Autodesk Fusion 360 part; units mm, degrees
(part 4 of 5)
sketch "Sketch1 (2)" plane through (0, 0, 25) normal (0, 0, 1) x (-1, 0, 0)
  arc A0 (-16.5263, 3.7625) -> (-16.7082, 2.8483) centre (0, 0) ccw
  arc A1 (-17.8062, 2.0227) -> (-16.7082, 2.8483) centre (-17.6939, 3.0163) ccw
  line L0 (-17.8062, 2.0227) -> (-18.6738, 2.1207)
  spline S0 degree 5 poles (-18.6738, 2.1207) (-18.6847, 2.1219) (-18.7065, 2.124) (-18.7393, 2.1263) (-18.783, 2.1276) (-18.8378, 2.1268) (-18.8928, 2.1242) (-18.9478, 2.1205) (-19.0028, 2.1162) (-19.0579, 2.1115) (-19.113, 2.1064) (-19.1681, 2.1008) (-19.2232, 2.0944) (-19.2784, 2.0871) (-19.3336, 2.079) (-19.3888, 2.0701) (-19.444, 2.0605) (-19.4992, 2.0503) (-19.5544, 2.0396) (-19.6096, 2.0285) (-19.6648, 2.0169) (-19.72, 2.0048) (-19.7752, 1.9921) (-19.8303, 1.9789) (-19.8855, 1.9652) (-19.9406, 1.9509) (-19.9957, 1.9362) (-20.0508, 1.921) (-20.1059, 1.9054) (-20.1609, 1.8893) (-20.2159, 1.8728) (-20.2709, 1.8558) (-20.3259, 1.8384) (-20.3808, 1.8206) (-20.4357, 1.8024) (-20.4906, 1.7837) (-20.5454, 1.7646) (-20.6002, 1.7451) (-20.655, 1.7252) (-20.7097, 1.7049) (-20.7643, 1.6842) (-20.819, 1.6631) (-20.8736, 1.6416) (-20.9281, 1.6198) (-20.9826, 1.5975) (-21.037, 1.5749) (-21.0914, 1.5519) (-21.1458, 1.5285) (-21.2001, 1.5048) (-21.2543, 1.4807) (-21.3085, 1.4563) (-21.3626, 1.4315) (-21.4167, 1.4063) (-21.4707, 1.3808) (-21.5247, 1.3549) (-21.5786, 1.3287) (-21.6324, 1.3021) (-21.6862, 1.2752) (-21.7399, 1.248) (-21.7936, 1.2204) (-21.8471, 1.1925) (-21.9007, 1.1642) (-21.9541, 1.1356) (-22.0075, 1.1067) (-22.0608, 1.0775) (-22.114, 1.0479) (-22.1672, 1.018) (-22.2203, 0.9878) (-22.2733, 0.9573) (-22.3263, 0.9265) (-22.3791, 0.8953) (-22.4214, 0.8701) (-22.453, 0.8511) (-22.4741, 0.8383) (-22.4846, 0.8319) knots 0 0 0 0 0 0 0.01428571 0.02857143 0.04285714 0.05714286 0.07142857 0.08571429 0.1 0.11428571 0.12857143 0.14285714 0.15714286 0.17142857 0.18571429 0.2 0.21428571 0.22857143 0.24285714 0.25714286 0.27142857 0.28571429 0.3 0.31428571 0.32857143 0.34285714 0.35714286 0.37142857 0.38571429 0.4 0.41428571 0.42857143 0.44285714 0.45714286 0.47142857 0.48571429 0.5 0.51428571 0.52857143 0.54285714 0.55714286 0.57142857 0.58571429 0.6 0.61428571 0.62857143 0.64285714 0.65714286 0.67142857 0.68571429 0.7 0.71428571 0.72857143 0.74285714 0.75714286 0.77142857 0.78571429 0.8 0.81428571 0.82857143 0.84285714 0.85714286 0.87142857 0.88571429 0.9 0.91428571 0.92857143 0.94285714 0.95714286 0.97142857 0.98571429 1 1 1 1 1 1
  arc A2 (-22.4846, 0.8319) -> (-22.4846, -0.8319) centre (0, 0) ccw
  spline S1 degree 5 poles (-22.4846, -0.8319) (-22.4741, -0.8383) (-22.453, -0.8511) (-22.4214, -0.8701) (-22.3791, -0.8953) (-22.3263, -0.9265) (-22.2733, -0.9573) (-22.2203, -0.9878) (-22.1672, -1.018) (-22.114, -1.0479) (-22.0608, -1.0775) (-22.0075, -1.1067) (-21.9541, -1.1356) (-21.9007, -1.1642) (-21.8471, -1.1925) (-21.7936, -1.2204) (-21.7399, -1.248) (-21.6862, -1.2752) (-21.6324, -1.3021) (-21.5786, -1.3287) (-21.5247, -1.3549) (-21.4707, -1.3808) (-21.4167, -1.4063) (-21.3626, -1.4315) (-21.3085, -1.4563) (-21.2543, -1.4807) (-21.2001, -1.5048) (-21.1458, -1.5285) (-21.0914, -1.5519) (-21.037, -1.5749) (-20.9826, -1.5975) (-20.9281, -1.6198) (-20.8736, -1.6416) (-20.819, -1.6631) (-20.7643, -1.6842) (-20.7097, -1.7049) (-20.655, -1.7252) (-20.6002, -1.7451) (-20.5454, -1.7646) (-20.4906, -1.7837) (-20.4357, -1.8024) (-20.3808, -1.8206) (-20.3259, -1.8384) (-20.2709, -1.8558) (-20.2159, -1.8728) (-20.1609, -1.8893) (-20.1059, -1.9054) (-20.0508, -1.921) (-19.9957, -1.9362) (-19.9406, -1.9509) (-19.8855, -1.9652) (-19.8303, -1.9789) (-19.7752, -1.9921) (-19.72, -2.0048) (-19.6648, -2.0169) (-19.6096, -2.0285) (-19.5544, -2.0396) (-19.4992, -2.0503) (-19.444, -2.0605) (-19.3888, -2.0701) (-19.3336, -2.079) (-19.2784, -2.0871) (-19.2232, -2.0944) (-19.1681, -2.1008) (-19.113, -2.1064) (-19.0579, -2.1115) (-19.0028, -2.1162) (-18.9478, -2.1205) (-18.8928, -2.1242) (-18.8378, -2.1268) (-18.783, -2.1276) (-18.7393, -2.1263) (-18.7065, -2.124) (-18.6847, -2.1219) (-18.6738, -2.1207) knots -1 -1 -1 -1 -1 -1 -0.98571429 -0.97142857 -0.95714286 -0.94285714 -0.92857143 -0.91428571 -0.9 -0.88571429 -0.87142857 -0.85714286 -0.84285714 -0.82857143 -0.81428571 -0.8 -0.78571429 -0.77142857 -0.75714286 -0.74285714 -0.72857143 -0.71428571 -0.7 -0.68571429 -0.67142857 -0.65714286 -0.64285714 -0.62857143 -0.61428571 -0.6 -0.58571429 -0.57142857 -0.55714286 -0.54285714 -0.52857143 -0.51428571 -0.5 -0.48571429 -0.47142857 -0.45714286 -0.44285714 -0.42857143 -0.41428571 -0.4 -0.38571429 -0.37142857 -0.35714286 -0.34285714 -0.32857143 -0.31428571 -0.3 -0.28571429 -0.27142857 -0.25714286 -0.24285714 -0.22857143 -0.21428571 -0.2 -0.18571429 -0.17142857 -0.15714286 -0.14285714 -0.12857143 -0.11428571 -0.1 -0.08571429 -0.07142857 -0.05714286 -0.04285714 -0.02857143 -0.01428571 0 0 0 0 0 0
  line L1 (-18.6738, -2.1207) -> (-17.8062, -2.0227)
  arc A3 (-16.7082, -2.8483) -> (-17.8062, -2.0227) centre (-17.6939, -3.0163) ccw
  arc A4 (-16.7082, -2.8483) -> (-16.5263, -3.7625) centre (0, 0) ccw
  arc A5 (-17.2248, -4.9454) -> (-16.5263, -3.7625) centre (-17.5014, -3.9844) ccw
  line L2 (-17.2248, -4.9454) -> (-18.0639, -5.1869)
  spline S2 degree 5 poles (-18.0639, -5.1869) (-18.0744, -5.19) (-18.0954, -5.1963) (-18.1265, -5.2067) (-18.1674, -5.2223) (-18.2178, -5.2441) (-18.2675, -5.2675) (-18.3169, -5.2919) (-18.3661, -5.3169) (-18.4152, -5.3423) (-18.4642, -5.3681) (-18.5129, -5.3944) (-18.5614, -5.4215) (-18.6096, -5.4493) (-18.6575, -5.4779) (-18.7051, -5.5073) (-18.7524, -5.5373) (-18.7995, -5.5678) (-18.8464, -5.5988) (-18.8932, -5.6302) (-18.9397, -5.662) (-18.9861, -5.6944) (-19.0322, -5.7272) (-19.0781, -5.7605) (-19.1238, -5.7942) (-19.1693, -5.8285) (-19.2146, -5.8632) (-19.2597, -5.8983) (-19.3046, -5.9338) (-19.3493, -5.9698) (-19.3938, -6.0061) (-19.4381, -6.0428) (-19.4822, -6.0799) (-19.5261, -6.1174) (-19.5699, -6.1552) (-19.6134, -6.1935) (-19.6568, -6.2321) (-19.6999, -6.2711) (-19.7429, -6.3105) (-19.7857, -6.3502) (-19.8283, -6.3902) (-19.8707, -6.4306) (-19.9129, -6.4713) (-19.9549, -6.5124) (-19.9967, -6.5538) (-20.0384, -6.5955) (-20.0798, -6.6376) (-20.1211, -6.68) (-20.1622, -6.7227) (-20.2031, -6.7657) (-20.2438, -6.809) (-20.2843, -6.8526) (-20.3246, -6.8966) (-20.3648, -6.9408) (-20.4047, -6.9854) (-20.4445, -7.0302) (-20.484, -7.0754) (-20.5234, -7.1208) (-20.5626, -7.1665) (-20.6016, -7.2125) (-20.6405, -7.2588) (-20.6791, -7.3054) (-20.7175, -7.3523) (-20.7558, -7.3994) (-20.7939, -7.4468) (-20.8317, -7.4945) (-20.8694, -7.5425) (-20.9069, -7.5907) (-20.9442, -7.6392) (-20.9813, -7.688) (-21.0182, -7.737) (-21.0476, -7.7764) (-21.0696, -7.8061) (-21.0842, -7.8259) (-21.0914, -7.8359) knots 0 0 0 0 0 0 0.01428571 0.02857143 0.04285714 0.05714286 0.07142857 0.08571429 0.1 0.11428571 0.12857143 0.14285714 0.15714286 0.17142857 0.18571429 0.2 0.21428571 0.22857143 0.24285714 0.25714286 0.27142857 0.28571429 0.3 0.31428571 0.32857143 0.34285714 0.35714286 0.37142857 0.38571429 0.4 0.41428571 0.42857143 0.44285714 0.45714286 0.47142857 0.48571429 0.5 0.51428571 0.52857143 0.54285714 0.55714286 0.57142857 0.58571429 0.6 0.61428571 0.62857143 0.64285714 0.65714286 0.67142857 0.68571429 0.7 0.71428571 0.72857143 0.74285714 0.75714286 0.77142857 0.78571429 0.8 0.81428571 0.82857143 0.84285714 0.85714286 0.87142857 0.88571429 0.9 0.91428571 0.92857143 0.94285714 0.95714286 0.97142857 0.98571429 1 1 1 1 1 1
  arc A6 (-21.0914, -7.8359) -> (-20.4547, -9.3731) centre (0, 0) ccw
  spline S3 degree 5 poles (-20.4547, -9.3731) (-20.4425, -9.375) (-20.4182, -9.3787) (-20.3817, -9.3842) (-20.333, -9.3913) (-20.2722, -9.3998) (-20.2115, -9.4081) (-20.1508, -9.416) (-20.0902, -9.4236) (-20.0297, -9.4308) (-19.9692, -9.4378) (-19.9087, -9.4444) (-19.8484, -9.4507) (-19.788, -9.4566) (-19.7278, -9.4622) (-19.6676, -9.4675) (-19.6075, -9.4725) (-19.5474, -9.4771) (-19.4874, -9.4814) (-19.4275, -9.4853) (-19.3677, -9.4889) (-19.308, -9.4922) (-19.2483, -9.4951) (-19.1887, -9.4976) (-19.1292, -9.4998) (-19.0698, -9.5017) (-19.0104, -9.5032) (-18.9512, -9.5043) (-18.8921, -9.5051) (-18.833, -9.5055) (-18.774, -9.5056) (-18.7152, -9.5053) (-18.6564, -9.5046) (-18.5978, -9.5036) (-18.5392, -9.5021) (-18.4808, -9.5003) (-18.4225, -9.4982) (-18.3643, -9.4956) (-18.3062, -9.4926) (-18.2482, -9.4893) (-18.1904, -9.4856) (-18.1327, -9.4814) (-18.0751, -9.4769) (-18.0177, -9.4719) (-17.9604, -9.4665) (-17.9033, -9.4607) (-17.8462, -9.4545) (-17.7894, -9.4479) (-17.7327, -9.4409) (-17.6761, -9.4334) (-17.6197, -9.4254) (-17.5635, -9.417) (-17.5075, -9.4081) (-17.4517, -9.3987) (-17.3961, -9.3887) (-17.3406, -9.3784) (-17.2854, -9.3675) (-17.2303, -9.3563) (-17.1754, -9.3445) (-17.1207, -9.3323) (-17.0663, -9.3194) (-17.0122, -9.3058) (-16.9585, -9.2914) (-16.9051, -9.2762) (-16.852, -9.2603) (-16.7991, -9.2439) (-16.7465, -9.2272) (-16.694, -9.2101) (-16.6417, -9.1924) (-16.59, -9.1738) (-16.539, -9.1536) (-16.4991, -9.1357) (-16.4697, -9.121) (-16.4504, -9.1107) (-16.4408, -9.1054) knots -1 -1 -1 -1 -1 -1 -0.98571429 -0.97142857 -0.95714286 -0.94285714 -0.92857143 -0.91428571 -0.9 -0.88571429 -0.87142857 -0.85714286 -0.84285714 -0.82857143 -0.81428571 -0.8 -0.78571429 -0.77142857 -0.75714286 -0.74285714 -0.72857143 -0.71428571 -0.7 -0.68571429 -0.67142857 -0.65714286 -0.64285714 -0.62857143 -0.61428571 -0.6 -0.58571429 -0.57142857 -0.55714286 -0.54285714 -0.52857143 -0.51428571 -0.5 -0.48571429 -0.47142857 -0.45714286 -0.44285714 -0.42857143 -0.41428571 -0.4 -0.38571429 -0.37142857 -0.35714286 -0.34285714 -0.32857143 -0.31428571 -0.3 -0.28571429 -0.27142857 -0.25714286 -0.24285714 -0.22857143 -0.21428571 -0.2 -0.18571429 -0.17142857 -0.15714286 -0.14285714 -0.12857143 -0.11428571 -0.1 -0.08571429 -0.07142857 -0.05714286 -0.04285714 -0.02857143 -0.01428571 0 0 0 0 0 0
  line L3 (-16.4408, -9.1054) -> (-15.6767, -8.6828)
  arc A7 (-14.3463, -9.0254) -> (-15.6767, -8.6828) centre (-15.1928, -9.5579) ccw
  arc A8 (-14.3463, -9.0254) -> (-13.8285, -9.8004) centre (0, 0) ccw
  arc A9 (-14.0211, -11.1606) -> (-13.8285, -9.8004) centre (-14.6444, -10.3786) ccw
  line L4 (-14.0211, -11.1606) -> (-14.7039, -11.7048)
  spline S4 degree 5 poles (-14.7039, -11.7048) (-14.7125, -11.7117) (-14.7294, -11.7256) (-14.7542, -11.7471) (-14.786, -11.7771) (-14.8242, -11.8165) (-14.8612, -11.8572) (-14.8975, -11.8987) (-14.9334, -11.9406) (-14.969, -11.9829) (-15.0044, -12.0254) (-15.0394, -12.0684) (-15.0738, -12.1119) (-15.1077, -12.1561) (-15.141, -12.2008) (-15.1737, -12.2462) (-15.206, -12.292) (-15.2378, -12.3382) (-15.2693, -12.3848) (-15.3004, -12.4317) (-15.3313, -12.479) (-15.3617, -12.5266) (-15.3918, -12.5745) (-15.4215, -12.6229) (-15.4507, -12.6716) (-15.4797, -12.7206) (-15.5082, -12.77) (-15.5364, -12.8197) (-15.5643, -12.8697) (-15.5919, -12.92) (-15.6191, -12.9706) (-15.646, -13.0214) (-15.6725, -13.0726) (-15.6988, -13.124) (-15.7247, -13.1758) (-15.7503, -13.2278) (-15.7755, -13.2801) (-15.8005, -13.3326) (-15.8251, -13.3854) (-15.8495, -13.4384) (-15.8735, -13.4917) (-15.8972, -13.5453) (-15.9206, -13.599) (-15.9437, -13.6531) (-15.9665, -13.7073) (-15.989, -13.7618) (-16.0113, -13.8165) (-16.0332, -13.8715) (-16.0548, -13.9267) (-16.0761, -13.982) (-16.0971, -14.0376) (-16.1179, -14.0935) (-16.1383, -14.1495) (-16.1584, -14.2057) (-16.1783, -14.2622) (-16.1979, -14.3188) (-16.2172, -14.3757) (-16.2362, -14.4327) (-16.2549, -14.49) (-16.2733, -14.5474) (-16.2915, -14.605) (-16.3093, -14.6629) (-16.3269, -14.7209) (-16.3442, -14.7791) (-16.3612, -14.8374) (-16.378, -14.896) (-16.3944, -14.9547) (-16.4106, -15.0136) (-16.4265, -15.0727) (-16.4421, -15.1319) (-16.4575, -15.1914) (-16.4696, -15.239) (-16.4785, -15.2749) (-16.4844, -15.2988) (-16.4873, -15.3108) knots 0 0 0 0 0 0 0.01428571 0.02857143 0.04285714 0.05714286 0.07142857 0.08571429 0.1 0.11428571 0.12857143 0.14285714 0.15714286 0.17142857 0.18571429 0.2 0.21428571 0.22857143 0.24285714 0.25714286 0.27142857 0.28571429 0.3 0.31428571 0.32857143 0.34285714 0.35714286 0.37142857 0.38571429 0.4 0.41428571 0.42857143 0.44285714 0.45714286 0.47142857 0.48571429 0.5 0.51428571 0.52857143 0.54285714 0.55714286 0.57142857 0.58571429 0.6 0.61428571 0.62857143 0.64285714 0.65714286 0.67142857 0.68571429 0.7 0.71428571 0.72857143 0.74285714 0.75714286 0.77142857 0.78571429 0.8 0.81428571 0.82857143 0.84285714 0.85714286 0.87142857 0.88571429 0.9 0.91428571 0.92857143 0.94285714 0.95714286 0.97142857 0.98571429 1 1 1 1 1 1
  arc A10 (-16.4873, -15.3108) -> (-15.3108, -16.4873) centre (0, 0) ccw
  spline S5 degree 5 poles (-15.3108, -16.4873) (-15.2988, -16.4844) (-15.2749, -16.4785) (-15.239, -16.4696) (-15.1914, -16.4575) (-15.1319, -16.4421) (-15.0727, -16.4265) (-15.0136, -16.4106) (-14.9547, -16.3944) (-14.896, -16.378) (-14.8374, -16.3612) (-14.7791, -16.3442) (-14.7209, -16.3269) (-14.6629, -16.3093) (-14.605, -16.2915) (-14.5474, -16.2733) (-14.49, -16.2549) (-14.4327, -16.2362) (-14.3757, -16.2172) (-14.3188, -16.1979) (-14.2622, -16.1783) (-14.2057, -16.1584) (-14.1495, -16.1383) (-14.0935, -16.1179) (-14.0376, -16.0971) (-13.982, -16.0761) (-13.9267, -16.0548) (-13.8715, -16.0332) (-13.8165, -16.0113) (-13.7618, -15.989) (-13.7073, -15.9665) (-13.6531, -15.9437) (-13.599, -15.9206) (-13.5453, -15.8972) (-13.4917, -15.8735) (-13.4384, -15.8495) (-13.3854, -15.8251) (-13.3326, -15.8005) (-13.2801, -15.7755) (-13.2278, -15.7503) (-13.1758, -15.7247) (-13.124, -15.6988) (-13.0726, -15.6725) (-13.0214, -15.646) (-12.9706, -15.6191) (-12.92, -15.5919) (-12.8697, -15.5643) (-12.8197, -15.5364) (-12.77, -15.5082) (-12.7206, -15.4797) (-12.6716, -15.4507) (-12.6229, -15.4215) (-12.5745, -15.3918) (-12.5266, -15.3617) (-12.479, -15.3313) (-12.4317, -15.3004) (-12.3848, -15.2693) (-12.3382, -15.2378) (-12.292, -15.206) (-12.2462, -15.1737) (-12.2008, -15.141) (-12.1561, -15.1077) (-12.1119, -15.0738) (-12.0684, -15.0394) (-12.0254, -15.0044) (-11.9829, -14.969) (-11.9406, -14.9334) (-11.8987, -14.8975) (-11.8572, -14.8612) (-11.8165, -14.8242) (-11.7771, -14.786) (-11.7471, -14.7542) (-11.7256, -14.7294) (-11.7117, -14.7125) (-11.7048, -14.7039) knots -1 -1 -1 -1 -1 -1 -0.98571429 -0.97142857 -0.95714286 -0.94285714 -0.92857143 -0.91428571 -0.9 -0.88571429 -0.87142857 -0.85714286 -0.84285714 -0.82857143 -0.81428571 -0.8 -0.78571429 -0.77142857 -0.75714286 -0.74285714 -0.72857143 -0.71428571 -0.7 -0.68571429 -0.67142857 -0.65714286 -0.64285714 -0.62857143 -0.61428571 -0.6 -0.58571429 -0.57142857 -0.55714286 -0.54285714 -0.52857143 -0.51428571 -0.5 -0.48571429 -0.47142857 -0.45714286 -0.44285714 -0.42857143 -0.41428571 -0.4 -0.38571429 -0.37142857 -0.35714286 -0.34285714 -0.32857143 -0.31428571 -0.3 -0.28571429 -0.27142857 -0.25714286 -0.24285714 -0.22857143 -0.21428571 -0.2 -0.18571429 -0.17142857 -0.15714286 -0.14285714 -0.12857143 -0.11428571 -0.1 -0.08571429 -0.07142857 -0.05714286 -0.04285714 -0.02857143 -0.01428571 0 0 0 0 0 0
  line L5 (-11.7048, -14.7039) -> (-11.1606, -14.0211)
  arc A11 (-9.8004, -13.8285) -> (-11.1606, -14.0211) centre (-10.3786, -14.6444) ccw
  arc A12 (-9.8004, -13.8285) -> (-9.0254, -14.3463) centre (0, 0) ccw
  arc A13 (-8.6828, -15.6767) -> (-9.0254, -14.3463) centre (-9.5579, -15.1928) ccw
  line L6 (-8.6828, -15.6767) -> (-9.1054, -16.4408)
  spline S6 degree 5 poles (-9.1054, -16.4408) (-9.1107, -16.4504) (-9.121, -16.4697) (-9.1357, -16.4991) (-9.1536, -16.539) (-9.1738, -16.59) (-9.1924, -16.6417) (-9.2101, -16.694) (-9.2272, -16.7465) (-9.2439, -16.7991) (-9.2603, -16.852) (-9.2762, -16.9051) (-9.2914, -16.9585) (-9.3058, -17.0122) (-9.3194, -17.0663) (-9.3323, -17.1207) (-9.3445, -17.1754) (-9.3563, -17.2303) (-9.3675, -17.2854) (-9.3784, -17.3406) (-9.3887, -17.3961) (-9.3987, -17.4517) (-9.4081, -17.5075) (-9.417, -17.5635) (-9.4254, -17.6197) (-9.4334, -17.6761) (-9.4409, -17.7327) (-9.4479, -17.7894) (-9.4545, -17.8462) (-9.4607, -17.9033) (-9.4665, -17.9604) (-9.4719, -18.0177) (-9.4769, -18.0751) (-9.4814, -18.1327) (-9.4856, -18.1904) (-9.4893, -18.2482) (-9.4926, -18.3062) (-9.4956, -18.3643) (-9.4982, -18.4225) (-9.5003, -18.4808) (-9.5021, -18.5392) (-9.5036, -18.5978) (-9.5046, -18.6564) (-9.5053, -18.7152) (-9.5056, -18.774) (-9.5055, -18.833) (-9.5051, -18.8921) (-9.5043, -18.9512) (-9.5032, -19.0104) (-9.5017, -19.0698) (-9.4998, -19.1292) (-9.4976, -19.1887) (-9.4951, -19.2483) (-9.4922, -19.308) (-9.4889, -19.3677) (-9.4853, -19.4275) (-9.4814, -19.4874) (-9.4771, -19.5474) (-9.4725, -19.6075) (-9.4675, -19.6676) (-9.4622, -19.7278) (-9.4566, -19.788) (-9.4507, -19.8484) (-9.4444, -19.9087) (-9.4378, -19.9692) (-9.4308, -20.0297) (-9.4236, -20.0902) (-9.416, -20.1508) (-9.4081, -20.2115) (-9.3998, -20.2722) (-9.3913, -20.333) (-9.3842, -20.3817) (-9.3787, -20.4182) (-9.375, -20.4425) (-9.3731, -20.4547) knots 0 0 0 0 0 0 0.01428571 0.02857143 0.04285714 0.05714286 0.07142857 0.08571429 0.1 0.11428571 0.12857143 0.14285714 0.15714286 0.17142857 0.18571429 0.2 0.21428571 0.22857143 0.24285714 0.25714286 0.27142857 0.28571429 0.3 0.31428571 0.32857143 0.34285714 0.35714286 0.37142857 0.38571429 0.4 0.41428571 0.42857143 0.44285714 0.45714286 0.47142857 0.48571429 0.5 0.51428571 0.52857143 0.54285714 0.55714286 0.57142857 0.58571429 0.6 0.61428571 0.62857143 0.64285714 0.65714286 0.67142857 0.68571429 0.7 0.71428571 0.72857143 0.74285714 0.75714286 0.77142857 0.78571429 0.8 0.81428571 0.82857143 0.84285714 0.85714286 0.87142857 0.88571429 0.9 0.91428571 0.92857143 0.94285714 0.95714286 0.97142857 0.98571429 1 1 1 1 1 1
  arc A14 (-9.3731, -20.4547) -> (-7.8359, -21.0914) centre (0, 0) ccw
  spline S7 degree 5 poles (-7.8359, -21.0914) (-7.8259, -21.0842) (-7.8061, -21.0696) (-7.7764, -21.0476) (-7.737, -21.0182) (-7.688, -20.9813) (-7.6392, -20.9442) (-7.5907, -20.9069) (-7.5425, -20.8694) (-7.4945, -20.8317) (-7.4468, -20.7939) (-7.3994, -20.7558) (-7.3523, -20.7175) (-7.3054, -20.6791) (-7.2588, -20.6405) (-7.2125, -20.6016) (-7.1665, -20.5626) (-7.1208, -20.5234) (-7.0754, -20.484) (-7.0302, -20.4445) (-6.9854, -20.4047) (-6.9408, -20.3648) (-6.8966, -20.3246) (-6.8526, -20.2843) (-6.809, -20.2438) (-6.7657, -20.2031) (-6.7227, -20.1622) (-6.68, -20.1211) (-6.6376, -20.0798) (-6.5955, -20.0384) (-6.5538, -19.9967) (-6.5124, -19.9549) (-6.4713, -19.9129) (-6.4306, -19.8707) (-6.3902, -19.8283) (-6.3502, -19.7857) (-6.3105, -19.7429) (-6.2711, -19.6999) (-6.2321, -19.6568) (-6.1935, -19.6134) (-6.1552, -19.5699) (-6.1174, -19.5261) (-6.0799, -19.4822) (-6.0428, -19.4381) (-6.0061, -19.3938) (-5.9698, -19.3493) (-5.9338, -19.3046) (-5.8983, -19.2597) (-5.8632, -19.2146) (-5.8285, -19.1693) (-5.7942, -19.1238) (-5.7605, -19.0781) (-5.7272, -19.0322) (-5.6944, -18.9861) (-5.662, -18.9397) (-5.6302, -18.8932) (-5.5988, -18.8464) (-5.5678, -18.7995) (-5.5373, -18.7524) (-5.5073, -18.7051) (-5.4779, -18.6575) (-5.4493, -18.6096) (-5.4215, -18.5614) (-5.3944, -18.5129) (-5.3681, -18.4642) (-5.3423, -18.4152) (-5.3169, -18.3661) (-5.2919, -18.3169) (-5.2675, -18.2675) (-5.2441, -18.2178) (-5.2223, -18.1674) (-5.2067, -18.1265) (-5.1963, -18.0954) (-5.19, -18.0744) (-5.1869, -18.0639) knots -1 -1 -1 -1 -1 -1 -0.98571429 -0.97142857 -0.95714286 -0.94285714 -0.92857143 -0.91428571 -0.9 -0.88571429 -0.87142857 -0.85714286 -0.84285714 -0.82857143 -0.81428571 -0.8 -0.78571429 -0.77142857 -0.75714286 -0.74285714 -0.72857143 -0.71428571 -0.7 -0.68571429 -0.67142857 -0.65714286 -0.64285714 -0.62857143 -0.61428571 -0.6 -0.58571429 -0.57142857 -0.55714286 -0.54285714 -0.52857143 -0.51428571 -0.5 -0.48571429 -0.47142857 -0.45714286 -0.44285714 -0.42857143 -0.41428571 -0.4 -0.38571429 -0.37142857 -0.35714286 -0.34285714 -0.32857143 -0.31428571 -0.3 -0.28571429 -0.27142857 -0.25714286 -0.24285714 -0.22857143 -0.21428571 -0.2 -0.18571429 -0.17142857 -0.15714286 -0.14285714 -0.12857143 -0.11428571 -0.1 -0.08571429 -0.07142857 -0.05714286 -0.04285714 -0.02857143 -0.01428571 0 0 0 0 0 0
  line L7 (-5.1869, -18.0639) -> (-4.9454, -17.2248)
  arc A15 (-3.7625, -16.5263) -> (-4.9454, -17.2248) centre (-3.9844, -17.5014) ccw
  arc A16 (-3.7625, -16.5263) -> (-2.8483, -16.7082) centre (0, 0) ccw
  arc A17 (-2.0227, -17.8062) -> (-2.8483, -16.7082) centre (-3.0163, -17.6939) ccw
  line L8 (-2.0227, -17.8062) -> (-2.1207, -18.6738)
  spline S8 degree 5 poles (-2.1207, -18.6738) (-2.1219, -18.6847) (-2.124, -18.7065) (-2.1263, -18.7393) (-2.1276, -18.783) (-2.1268, -18.8378) (-2.1242, -18.8928) (-2.1205, -18.9478) (-2.1162, -19.0028) (-2.1115, -19.0579) (-2.1064, -19.113) (-2.1008, -19.1681) (-2.0944, -19.2232) (-2.0871, -19.2784) (-2.079, -19.3336) (-2.0701, -19.3888) (-2.0605, -19.444) (-2.0503, -19.4992) (-2.0396, -19.5544) (-2.0285, -19.6096) (-2.0169, -19.6648) (-2.0048, -19.72) (-1.9921, -19.7752) (-1.9789, -19.8303) (-1.9652, -19.8855) (-1.9509, -19.9406) (-1.9362, -19.9957) (-1.921, -20.0508) (-1.9054, -20.1059) (-1.8893, -20.1609) (-1.8728, -20.2159) (-1.8558, -20.2709) (-1.8384, -20.3259) (-1.8206, -20.3808) (-1.8024, -20.4357) (-1.7837, -20.4906) (-1.7646, -20.5454) (-1.7451, -20.6002) (-1.7252, -20.655) (-1.7049, -20.7097) (-1.6842, -20.7643) (-1.6631, -20.819) (-1.6416, -20.8736) (-1.6198, -20.9281) (-1.5975, -20.9826) (-1.5749, -21.037) (-1.5519, -21.0914) (-1.5285, -21.1458) (-1.5048, -21.2001) (-1.4807, -21.2543) (-1.4563, -21.3085) (-1.4315, -21.3626) (-1.4063, -21.4167) (-1.3808, -21.4707) (-1.3549, -21.5247) (-1.3287, -21.5786) (-1.3021, -21.6324) (-1.2752, -21.6862) (-1.248, -21.7399) (-1.2204, -21.7936) (-1.1925, -21.8471) (-1.1642, -21.9007) (-1.1356, -21.9541) (-1.1067, -22.0075) (-1.0775, -22.0608) (-1.0479, -22.114) (-1.018, -22.1672) (-0.9878, -22.2203) (-0.9573, -22.2733) (-0.9265, -22.3263) (-0.8953, -22.3791) (-0.8701, -22.4214) (-0.8511, -22.453) (-0.8383, -22.4741) (-0.8319, -22.4846) knots 0 0 0 0 0 0 0.01428571 0.02857143 0.04285714 0.05714286 0.07142857 0.08571429 0.1 0.11428571 0.12857143 0.14285714 0.15714286 0.17142857 0.18571429 0.2 0.21428571 0.22857143 0.24285714 0.25714286 0.27142857 0.28571429 0.3 0.31428571 0.32857143 0.34285714 0.35714286 0.37142857 0.38571429 0.4 0.41428571 0.42857143 0.44285714 0.45714286 0.47142857 0.48571429 0.5 0.51428571 0.52857143 0.54285714 0.55714286 0.57142857 0.58571429 0.6 0.61428571 0.62857143 0.64285714 0.65714286 0.67142857 0.68571429 0.7 0.71428571 0.72857143 0.74285714 0.75714286 0.77142857 0.78571429 0.8 0.81428571 0.82857143 0.84285714 0.85714286 0.87142857 0.88571429 0.9 0.91428571 0.92857143 0.94285714 0.95714286 0.97142857 0.98571429 1 1 1 1 1 1
  arc A18 (-0.8319, -22.4846) -> (0.8319, -22.4846) centre (0, 0) ccw
  spline S9 degree 5 poles (0.8319, -22.4846) (0.8383, -22.4741) (0.8511, -22.453) (0.8701, -22.4214) (0.8953, -22.3791) (0.9265, -22.3263) (0.9573, -22.2733) (0.9878, -22.2203) (1.018, -22.1672) (1.0479, -22.114) (1.0775, -22.0608) (1.1067, -22.0075) (1.1356, -21.9541) (1.1642, -21.9007) (1.1925, -21.8471) (1.2204, -21.7936) (1.248, -21.7399) (1.2752, -21.6862) (1.3021, -21.6324) (1.3287, -21.5786) (1.3549, -21.5247) (1.3808, -21.4707) (1.4063, -21.4167) (1.4315, -21.3626) (1.4563, -21.3085) (1.4807, -21.2543) (1.5048, -21.2001) (1.5285, -21.1458) (1.5519, -21.0914) (1.5749, -21.037) (1.5975, -20.9826) (1.6198, -20.9281) (1.6416, -20.8736) (1.6631, -20.819) (1.6842, -20.7643) (1.7049, -20.7097) (1.7252, -20.655) (1.7451, -20.6002) (1.7646, -20.5454) (1.7837, -20.4906) (1.8024, -20.4357) (1.8206, -20.3808) (1.8384, -20.3259) (1.8558, -20.2709) (1.8728, -20.2159) (1.8893, -20.1609) (1.9054, -20.1059) (1.921, -20.0508) (1.9362, -19.9957) (1.9509, -19.9406) (1.9652, -19.8855) (1.9789, -19.8303) (1.9921, -19.7752) (2.0048, -19.72) (2.0169, -19.6648) (2.0285, -19.6096) (2.0396, -19.5544) (2.0503, -19.4992) (2.0605, -19.444) (2.0701, -19.3888) (2.079, -19.3336) (2.0871, -19.2784) (2.0944, -19.2232) (2.1008, -19.1681) (2.1064, -19.113) (2.1115, -19.0579) (2.1162, -19.0028) (2.1205, -18.9478) (2.1242, -18.8928) (2.1268, -18.8378) (2.1276, -18.783) (2.1263, -18.7393) (2.124, -18.7065) (2.1219, -18.6847) (2.1207, -18.6738) knots -1 -1 -1 -1 -1 -1 -0.98571429 -0.97142857 -0.95714286 -0.94285714 -0.92857143 -0.91428571 -0.9 -0.88571429 -0.87142857 -0.85714286 -0.84285714 -0.82857143 -0.81428571 -0.8 -0.78571429 -0.77142857 -0.75714286 -0.74285714 -0.72857143 -0.71428571 -0.7 -0.68571429 -0.67142857 -0.65714286 -0.64285714 -0.62857143 -0.61428571 -0.6 -0.58571429 -0.57142857 -0.55714286 -0.54285714 -0.52857143 -0.51428571 -0.5 -0.48571429 -0.47142857 -0.45714286 -0.44285714 -0.42857143 -0.41428571 -0.4 -0.38571429 -0.37142857 -0.35714286 -0.34285714 -0.32857143 -0.31428571 -0.3 -0.28571429 -0.27142857 -0.25714286 -0.24285714 -0.22857143 -0.21428571 -0.2 -0.18571429 -0.17142857 -0.15714286 -0.14285714 -0.12857143 -0.11428571 -0.1 -0.08571429 -0.07142857 -0.05714286 -0.04285714 -0.02857143 -0.01428571 0 0 0 0 0 0
  line L9 (2.1207, -18.6738) -> (2.0227, -17.8062)
  arc A19 (2.8483, -16.7082) -> (2.0227, -17.8062) centre (3.0163, -17.6939) ccw
  arc A20 (2.8483, -16.7082) -> (3.7625, -16.5263) centre (0, 0) ccw
  arc A21 (4.9454, -17.2248) -> (3.7625, -16.5263) centre (3.9844, -17.5014) ccw
  line L10 (4.9454, -17.2248) -> (5.1869, -18.0639)
  spline S10 degree 5 poles (5.1869, -18.0639) (5.19, -18.0744) (5.1963, -18.0954) (5.2067, -18.1265) (5.2223, -18.1674) (5.2441, -18.2178) (5.2675, -18.2675) (5.2919, -18.3169) (5.3169, -18.3661) (5.3423, -18.4152) (5.3681, -18.4642) (5.3944, -18.5129) (5.4215, -18.5614) (5.4493, -18.6096) (5.4779, -18.6575) (5.5073, -18.7051) (5.5373, -18.7524) (5.5678, -18.7995) (5.5988, -18.8464) (5.6302, -18.8932) (5.662, -18.9397) (5.6944, -18.9861) (5.7272, -19.0322) (5.7605, -19.0781) (5.7942, -19.1238) (5.8285, -19.1693) (5.8632, -19.2146) (5.8983, -19.2597) (5.9338, -19.3046) (5.9698, -19.3493) (6.0061, -19.3938) (6.0428, -19.4381) (6.0799, -19.4822) (6.1174, -19.5261) (6.1552, -19.5699) (6.1935, -19.6134) (6.2321, -19.6568) (6.2711, -19.6999) (6.3105, -19.7429) (6.3502, -19.7857) (6.3902, -19.8283) (6.4306, -19.8707) (6.4713, -19.9129) (6.5124, -19.9549) (6.5538, -19.9967) (6.5955, -20.0384) (6.6376, -20.0798) (6.68, -20.1211) (6.7227, -20.1622) (6.7657, -20.2031) (6.809, -20.2438) (6.8526, -20.2843) (6.8966, -20.3246) (6.9408, -20.3648) (6.9854, -20.4047) (7.0302, -20.4445) (7.0754, -20.484) (7.1208, -20.5234) (7.1665, -20.5626) (7.2125, -20.6016) (7.2588, -20.6405) (7.3054, -20.6791) (7.3523, -20.7175) (7.3994, -20.7558) (7.4468, -20.7939) (7.4945, -20.8317) (7.5425, -20.8694) (7.5907, -20.9069) (7.6392, -20.9442) (7.688, -20.9813) (7.737, -21.0182) (7.7764, -21.0476) (7.8061, -21.0696) (7.8259, -21.0842) (7.8359, -21.0914) knots 0 0 0 0 0 0 0.01428571 0.02857143 0.04285714 0.05714286 0.07142857 0.08571429 0.1 0.11428571 0.12857143 0.14285714 0.15714286 0.17142857 0.18571429 0.2 0.21428571 0.22857143 0.24285714 0.25714286 0.27142857 0.28571429 0.3 0.31428571 0.32857143 0.34285714 0.35714286 0.37142857 0.38571429 0.4 0.41428571 0.42857143 0.44285714 0.45714286 0.47142857 0.48571429 0.5 0.51428571 0.52857143 0.54285714 0.55714286 0.57142857 0.58571429 0.6 0.61428571 0.62857143 0.64285714 0.65714286 0.67142857 0.68571429 0.7 0.71428571 0.72857143 0.74285714 0.75714286 0.77142857 0.78571429 0.8 0.81428571 0.82857143 0.84285714 0.85714286 0.87142857 0.88571429 0.9 0.91428571 0.92857143 0.94285714 0.95714286 0.97142857 0.98571429 1 1 1 1 1 1
  arc A22 (7.8359, -21.0914) -> (9.3731, -20.4547) centre (0, 0) ccw
  spline S11 degree 5 poles (9.3731, -20.4547) (9.375, -20.4425) (9.3787, -20.4182) (9.3842, -20.3817) (9.3913, -20.333) (9.3998, -20.2722) (9.4081, -20.2115) (9.416, -20.1508) (9.4236, -20.0902) (9.4308, -20.0297) (9.4378, -19.9692) (9.4444, -19.9087) (9.4507, -19.8484) (9.4566, -19.788) (9.4622, -19.7278) (9.4675, -19.6676) (9.4725, -19.6075) (9.4771, -19.5474) (9.4814, -19.4874) (9.4853, -19.4275) (9.4889, -19.3677) (9.4922, -19.308) (9.4951, -19.2483) (9.4976, -19.1887) (9.4998, -19.1292) (9.5017, -19.0698) (9.5032, -19.0104) (9.5043, -18.9512) (9.5051, -18.8921) (9.5055, -18.833) (9.5056, -18.774) (9.5053, -18.7152) (9.5046, -18.6564) (9.5036, -18.5978) (9.5021, -18.5392) (9.5003, -18.4808) (9.4982, -18.4225) (9.4956, -18.3643) (9.4926, -18.3062) (9.4893, -18.2482) (9.4856, -18.1904) (9.4814, -18.1327) (9.4769, -18.0751) (9.4719, -18.0177) (9.4665, -17.9604) (9.4607, -17.9033) (9.4545, -17.8462) (9.4479, -17.7894) (9.4409, -17.7327) (9.4334, -17.6761) (9.4254, -17.6197) (9.417, -17.5635) (9.4081, -17.5075) (9.3987, -17.4517) (9.3887, -17.3961) (9.3784, -17.3406) (9.3675, -17.2854) (9.3563, -17.2303) (9.3445, -17.1754) (9.3323, -17.1207) (9.3194, -17.0663) (9.3058, -17.0122) (9.2914, -16.9585) (9.2762, -16.9051) (9.2603, -16.852) (9.2439, -16.7991) (9.2272, -16.7465) (9.2101, -16.694) (9.1924, -16.6417) (9.1738, -16.59) (9.1536, -16.539) (9.1357, -16.4991) (9.121, -16.4697) (9.1107, -16.4504) (9.1054, -16.4408) knots -1 -1 -1 -1 -1 -1 -0.98571429 -0.97142857 -0.95714286 -0.94285714 -0.92857143 -0.91428571 -0.9 -0.88571429 -0.87142857 -0.85714286 -0.84285714 -0.82857143 -0.81428571 -0.8 -0.78571429 -0.77142857 -0.75714286 -0.74285714 -0.72857143 -0.71428571 -0.7 -0.68571429 -0.67142857 -0.65714286 -0.64285714 -0.62857143 -0.61428571 -0.6 -0.58571429 -0.57142857 -0.55714286 -0.54285714 -0.52857143 -0.51428571 -0.5 -0.48571429 -0.47142857 -0.45714286 -0.44285714 -0.42857143 -0.41428571 -0.4 -0.38571429 -0.37142857 -0.35714286 -0.34285714 -0.32857143 -0.31428571 -0.3 -0.28571429 -0.27142857 -0.25714286 -0.24285714 -0.22857143 -0.21428571 -0.2 -0.18571429 -0.17142857 -0.15714286 -0.14285714 -0.12857143 -0.11428571 -0.1 -0.08571429 -0.07142857 -0.05714286 -0.04285714 -0.02857143 -0.01428571 0 0 0 0 0 0
  line L11 (9.1054, -16.4408) -> (8.6828, -15.6767)
  arc A23 (9.0254, -14.3463) -> (8.6828, -15.6767) centre (9.5579, -15.1928) ccw
  arc A24 (9.0254, -14.3463) -> (9.8004, -13.8285) centre (0, 0) ccw
  arc A25 (11.1606, -14.0211) -> (9.8004, -13.8285) centre (10.3786, -14.6444) ccw
  line L12 (11.1606, -14.0211) -> (11.7048, -14.7039)
  spline S12 degree 5 poles (11.7048, -14.7039) (11.7117, -14.7125) (11.7256, -14.7294) (11.7471, -14.7542) (11.7771, -14.786) (11.8165, -14.8242) (11.8572, -14.8612) (11.8987, -14.8975) (11.9406, -14.9334) (11.9829, -14.969) (12.0254, -15.0044) (12.0684, -15.0394) (12.1119, -15.0738) (12.1561, -15.1077) (12.2008, -15.141) (12.2462, -15.1737) (12.292, -15.206) (12.3382, -15.2378) (12.3848, -15.2693) (12.4317, -15.3004) (12.479, -15.3313) (12.5266, -15.3617) (12.5745, -15.3918) (12.6229, -15.4215) (12.6716, -15.4507) (12.7206, -15.4797) (12.77, -15.5082) (12.8197, -15.5364) (12.8697, -15.5643) (12.92, -15.5919) (12.9706, -15.6191) (13.0214, -15.646) (13.0726, -15.6725) (13.124, -15.6988) (13.1758, -15.7247) (13.2278, -15.7503) (13.2801, -15.7755) (13.3326, -15.8005) (13.3854, -15.8251) (13.4384, -15.8495) (13.4917, -15.8735) (13.5453, -15.8972) (13.599, -15.9206) (13.6531, -15.9437) (13.7073, -15.9665) (13.7618, -15.989) (13.8165, -16.0113) (13.8715, -16.0332) (13.9267, -16.0548) (13.982, -16.0761) (14.0376, -16.0971) (14.0935, -16.1179) (14.1495, -16.1383) (14.2057, -16.1584) (14.2622, -16.1783) (14.3188, -16.1979) (14.3757, -16.2172) (14.4327, -16.2362) (14.49, -16.2549) (14.5474, -16.2733) (14.605, -16.2915) (14.6629, -16.3093) (14.7209, -16.3269) (14.7791, -16.3442) (14.8374, -16.3612) (14.896, -16.378) (14.9547, -16.3944) (15.0136, -16.4106) (15.0727, -16.4265) (15.1319, -16.4421) (15.1914, -16.4575) (15.239, -16.4696) (15.2749, -16.4785) (15.2988, -16.4844) (15.3108, -16.4873) knots 0 0 0 0 0 0 0.01428571 0.02857143 0.04285714 0.05714286 0.07142857 0.08571429 0.1 0.11428571 0.12857143 0.14285714 0.15714286 0.17142857 0.18571429 0.2 0.21428571 0.22857143 0.24285714 0.25714286 0.27142857 0.28571429 0.3 0.31428571 0.32857143 0.34285714 0.35714286 0.37142857 0.38571429 0.4 0.41428571 0.42857143 0.44285714 0.45714286 0.47142857 0.48571429 0.5 0.51428571 0.52857143 0.54285714 0.55714286 0.57142857 0.58571429 0.6 0.61428571 0.62857143 0.64285714 0.65714286 0.67142857 0.68571429 0.7 0.71428571 0.72857143 0.74285714 0.75714286 0.77142857 0.78571429 0.8 0.81428571 0.82857143 0.84285714 0.85714286 0.87142857 0.88571429 0.9 0.91428571 0.92857143 0.94285714 0.95714286 0.97142857 0.98571429 1 1 1 1 1 1
  arc A26 (15.3108, -16.4873) -> (16.4873, -15.3108) centre (0, 0) ccw
  spline S13 degree 5 poles (16.4873, -15.3108) (16.4844, -15.2988) (16.4785, -15.2749) (16.4696, -15.239) (16.4575, -15.1914) (16.4421, -15.1319) (16.4265, -15.0727) (16.4106, -15.0136) (16.3944, -14.9547) (16.378, -14.896) (16.3612, -14.8374) (16.3442, -14.7791) (16.3269, -14.7209) (16.3093, -14.6629) (16.2915, -14.605) (16.2733, -14.5474) (16.2549, -14.49) (16.2362, -14.4327) (16.2172, -14.3757) (16.1979, -14.3188) (16.1783, -14.2622) (16.1584, -14.2057) (16.1383, -14.1495) (16.1179, -14.0935) (16.0971, -14.0376) (16.0761, -13.982) (16.0548, -13.9267) (16.0332, -13.8715) (16.0113, -13.8165) (15.989, -13.7618) (15.9665, -13.7073) (15.9437, -13.6531) (15.9206, -13.599) (15.8972, -13.5453) (15.8735, -13.4917) (15.8495, -13.4384) (15.8251, -13.3854) (15.8005, -13.3326) (15.7755, -13.2801) (15.7503, -13.2278) (15.7247, -13.1758) (15.6988, -13.124) (15.6725, -13.0726) (15.646, -13.0214) (15.6191, -12.9706) (15.5919, -12.92) (15.5643, -12.8697) (15.5364, -12.8197) (15.5082, -12.77) (15.4797, -12.7206) (15.4507, -12.6716) (15.4215, -12.6229) (15.3918, -12.5745) (15.3617, -12.5266) (15.3313, -12.479) (15.3004, -12.4317) (15.2693, -12.3848) (15.2378, -12.3382) (15.206, -12.292) (15.1737, -12.2462) (15.141, -12.2008) (15.1077, -12.1561) (15.0738, -12.1119) (15.0394, -12.0684) (15.0044, -12.0254) (14.969, -11.9829) (14.9334, -11.9406) (14.8975, -11.8987) (14.8612, -11.8572) (14.8242, -11.8165) (14.786, -11.7771) (14.7542, -11.7471) (14.7294, -11.7256) (14.7125, -11.7117) (14.7039, -11.7048) knots -1 -1 -1 -1 -1 -1 -0.98571429 -0.97142857 -0.95714286 -0.94285714 -0.92857143 -0.91428571 -0.9 -0.88571429 -0.87142857 -0.85714286 -0.84285714 -0.82857143 -0.81428571 -0.8 -0.78571429 -0.77142857 -0.75714286 -0.74285714 -0.72857143 -0.71428571 -0.7 -0.68571429 -0.67142857 -0.65714286 -0.64285714 -0.62857143 -0.61428571 -0.6 -0.58571429 -0.57142857 -0.55714286 -0.54285714 -0.52857143 -0.51428571 -0.5 -0.48571429 -0.47142857 -0.45714286 -0.44285714 -0.42857143 -0.41428571 -0.4 -0.38571429 -0.37142857 -0.35714286 -0.34285714 -0.32857143 -0.31428571 -0.3 -0.28571429 -0.27142857 -0.25714286 -0.24285714 -0.22857143 -0.21428571 -0.2 -0.18571429 -0.17142857 -0.15714286 -0.14285714 -0.12857143 -0.11428571 -0.1 -0.08571429 -0.07142857 -0.05714286 -0.04285714 -0.02857143 -0.01428571 0 0 0 0 0 0
  line L13 (14.7039, -11.7048) -> (14.0211, -11.1606)
  arc A27 (13.8285, -9.8004) -> (14.0211, -11.1606) centre (14.6444, -10.3786) ccw
  arc A28 (13.8285, -9.8004) -> (14.3463, -9.0254) centre (0, 0) ccw
  arc A29 (15.6767, -8.6828) -> (14.3463, -9.0254) centre (15.1928, -9.5579) ccw
  line L14 (15.6767, -8.6828) -> (16.4408, -9.1054)
  spline S14 degree 5 poles (16.4408, -9.1054) (16.4504, -9.1107) (16.4697, -9.121) (16.4991, -9.1357) (16.539, -9.1536) (16.59, -9.1738) (16.6417, -9.1924) (16.694, -9.2101) (16.7465, -9.2272) (16.7991, -9.2439) (16.852, -9.2603) (16.9051, -9.2762) (16.9585, -9.2914) (17.0122, -9.3058) (17.0663, -9.3194) (17.1207, -9.3323) (17.1754, -9.3445) (17.2303, -9.3563) (17.2854, -9.3675) (17.3406, -9.3784) (17.3961, -9.3887) (17.4517, -9.3987) (17.5075, -9.4081) (17.5635, -9.417) (17.6197, -9.4254) (17.6761, -9.4334) (17.7327, -9.4409) (17.7894, -9.4479) (17.8462, -9.4545) (17.9033, -9.4607) (17.9604, -9.4665) (18.0177, -9.4719) (18.0751, -9.4769) (18.1327, -9.4814) (18.1904, -9.4856) (18.2482, -9.4893) (18.3062, -9.4926) (18.3643, -9.4956) (18.4225, -9.4982) (18.4808, -9.5003) (18.5392, -9.5021) (18.5978, -9.5036) (18.6564, -9.5046) (18.7152, -9.5053) (18.774, -9.5056) (18.833, -9.5055) (18.8921, -9.5051) (18.9512, -9.5043) (19.0104, -9.5032) (19.0698, -9.5017) (19.1292, -9.4998) (19.1887, -9.4976) (19.2483, -9.4951) (19.308, -9.4922) (19.3677, -9.4889) (19.4275, -9.4853) (19.4874, -9.4814) (19.5474, -9.4771) (19.6075, -9.4725) (19.6676, -9.4675) (19.7278, -9.4622) (19.788, -9.4566) (19.8484, -9.4507) (19.9087, -9.4444) (19.9692, -9.4378) (20.0297, -9.4308) (20.0902, -9.4236) (20.1508, -9.416) (20.2115, -9.4081) (20.2722, -9.3998) (20.333, -9.3913) (20.3817, -9.3842) (20.4182, -9.3787) (20.4425, -9.375) (20.4547, -9.3731) knots 0 0 0 0 0 0 0.01428571 0.02857143 0.04285714 0.05714286 0.07142857 0.08571429 0.1 0.11428571 0.12857143 0.14285714 0.15714286 0.17142857 0.18571429 0.2 0.21428571 0.22857143 0.24285714 0.25714286 0.27142857 0.28571429 0.3 0.31428571 0.32857143 0.34285714 0.35714286 0.37142857 0.38571429 0.4 0.41428571 0.42857143 0.44285714 0.45714286 0.47142857 0.48571429 0.5 0.51428571 0.52857143 0.54285714 0.55714286 0.57142857 0.58571429 0.6 0.61428571 0.62857143 0.64285714 0.65714286 0.67142857 0.68571429 0.7 0.71428571 0.72857143 0.74285714 0.75714286 0.77142857 0.78571429 0.8 0.81428571 0.82857143 0.84285714 0.85714286 0.87142857 0.88571429 0.9 0.91428571 0.92857143 0.94285714 0.95714286 0.97142857 0.98571429 1 1 1 1 1 1
  arc A30 (20.4547, -9.3731) -> (21.0914, -7.8359) centre (0, 0) ccw
  spline S15 degree 5 poles (21.0914, -7.8359) (21.0842, -7.8259) (21.0696, -7.8061) (21.0476, -7.7764) (21.0182, -7.737) (20.9813, -7.688) (20.9442, -7.6392) (20.9069, -7.5907) (20.8694, -7.5425) (20.8317, -7.4945) (20.7939, -7.4468) (20.7558, -7.3994) (20.7175, -7.3523) (20.6791, -7.3054) (20.6405, -7.2588) (20.6016, -7.2125) (20.5626, -7.1665) (20.5234, -7.1208) (20.484, -7.0754) (20.4445, -7.0302) (20.4047, -6.9854) (20.3648, -6.9408) (20.3246, -6.8966) (20.2843, -6.8526) (20.2438, -6.809) (20.2031, -6.7657) (20.1622, -6.7227) (20.1211, -6.68) (20.0798, -6.6376) (20.0384, -6.5955) (19.9967, -6.5538) (19.9549, -6.5124) (19.9129, -6.4713) (19.8707, -6.4306) (19.8283, -6.3902) (19.7857, -6.3502) (19.7429, -6.3105) (19.6999, -6.2711) (19.6568, -6.2321) (19.6134, -6.1935) (19.5699, -6.1552) (19.5261, -6.1174) (19.4822, -6.0799) (19.4381, -6.0428) (19.3938, -6.0061) (19.3493, -5.9698) (19.3046, -5.9338) (19.2597, -5.8983) (19.2146, -5.8632) (19.1693, -5.8285) (19.1238, -5.7942) (19.0781, -5.7605) (19.0322, -5.7272) (18.9861, -5.6944) (18.9397, -5.662) (18.8932, -5.6302) (18.8464, -5.5988) (18.7995, -5.5678) (18.7524, -5.5373) (18.7051, -5.5073) (18.6575, -5.4779) (18.6096, -5.4493) (18.5614, -5.4215) (18.5129, -5.3944) (18.4642, -5.3681) (18.4152, -5.3423) (18.3661, -5.3169) (18.3169, -5.2919) (18.2675, -5.2675) (18.2178, -5.2441) (18.1674, -5.2223) (18.1265, -5.2067) (18.0954, -5.1963) (18.0744, -5.19) (18.0639, -5.1869) knots -1 -1 -1 -1 -1 -1 -0.98571429 -0.97142857 -0.95714286 -0.94285714 -0.92857143 -0.91428571 -0.9 -0.88571429 -0.87142857 -0.85714286 -0.84285714 -0.82857143 -0.81428571 -0.8 -0.78571429 -0.77142857 -0.75714286 -0.74285714 -0.72857143 -0.71428571 -0.7 -0.68571429 -0.67142857 -0.65714286 -0.64285714 -0.62857143 -0.61428571 -0.6 -0.58571429 -0.57142857 -0.55714286 -0.54285714 -0.52857143 -0.51428571 -0.5 -0.48571429 -0.47142857 -0.45714286 -0.44285714 -0.42857143 -0.41428571 -0.4 -0.38571429 -0.37142857 -0.35714286 -0.34285714 -0.32857143 -0.31428571 -0.3 -0.28571429 -0.27142857 -0.25714286 -0.24285714 -0.22857143 -0.21428571 -0.2 -0.18571429 -0.17142857 -0.15714286 -0.14285714 -0.12857143 -0.11428571 -0.1 -0.08571429 -0.07142857 -0.05714286 -0.04285714 -0.02857143 -0.01428571 0 0 0 0 0 0
  line L15 (18.0639, -5.1869) -> (17.2248, -4.9454)
  arc A31 (16.5263, -3.7625) -> (17.2248, -4.9454) centre (17.5014, -3.9844) ccw
  arc A32 (16.5263, -3.7625) -> (16.7082, -2.8483) centre (0, 0) ccw
  arc A33 (17.8062, -2.0227) -> (16.7082, -2.8483) centre (17.6939, -3.0163) ccw
  line L16 (17.8062, -2.0227) -> (18.6738, -2.1207)
  spline S16 degree 5 poles (18.6738, -2.1207) (18.6847, -2.1219) (18.7065, -2.124) (18.7393, -2.1263) (18.783, -2.1276) (18.8378, -2.1268) (18.8928, -2.1242) (18.9478, -2.1205) (19.0028, -2.1162) (19.0579, -2.1115) (19.113, -2.1064) (19.1681, -2.1008) (19.2232, -2.0944) (19.2784, -2.0871) (19.3336, -2.079) (19.3888, -2.0701) (19.444, -2.0605) (19.4992, -2.0503) (19.5544, -2.0396) (19.6096, -2.0285) (19.6648, -2.0169) (19.72, -2.0048) (19.7752, -1.9921) (19.8303, -1.9789) (19.8855, -1.9652) (19.9406, -1.9509) (19.9957, -1.9362) (20.0508, -1.921) (20.1059, -1.9054) (20.1609, -1.8893) (20.2159, -1.8728) (20.2709, -1.8558) (20.3259, -1.8384) (20.3808, -1.8206) (20.4357, -1.8024) (20.4906, -1.7837) (20.5454, -1.7646) (20.6002, -1.7451) (20.655, -1.7252) (20.7097, -1.7049) (20.7643, -1.6842) (20.819, -1.6631) (20.8736, -1.6416) (20.9281, -1.6198) (20.9826, -1.5975) (21.037, -1.5749) (21.0914, -1.5519) (21.1458, -1.5285) (21.2001, -1.5048) (21.2543, -1.4807) (21.3085, -1.4563) (21.3626, -1.4315) (21.4167, -1.4063) (21.4707, -1.3808) (21.5247, -1.3549) (21.5786, -1.3287) (21.6324, -1.3021) (21.6862, -1.2752) (21.7399, -1.248) (21.7936, -1.2204) (21.8471, -1.1925) (21.9007, -1.1642) (21.9541, -1.1356) (22.0075, -1.1067) (22.0608, -1.0775) (22.114, -1.0479) (22.1672, -1.018) (22.2203, -0.9878) (22.2733, -0.9573) (22.3263, -0.9265) (22.3791, -0.8953) (22.4214, -0.8701) (22.453, -0.8511) (22.4741, -0.8383) (22.4846, -0.8319) knots 0 0 0 0 0 0 0.01428571 0.02857143 0.04285714 0.05714286 0.07142857 0.08571429 0.1 0.11428571 0.12857143 0.14285714 0.15714286 0.17142857 0.18571429 0.2 0.21428571 0.22857143 0.24285714 0.25714286 0.27142857 0.28571429 0.3 0.31428571 0.32857143 0.34285714 0.35714286 0.37142857 0.38571429 0.4 0.41428571 0.42857143 0.44285714 0.45714286 0.47142857 0.48571429 0.5 0.51428571 0.52857143 0.54285714 0.55714286 0.57142857 0.58571429 0.6 0.61428571 0.62857143 0.64285714 0.65714286 0.67142857 0.68571429 0.7 0.71428571 0.72857143 0.74285714 0.75714286 0.77142857 0.78571429 0.8 0.81428571 0.82857143 0.84285714 0.85714286 0.87142857 0.88571429 0.9 0.91428571 0.92857143 0.94285714 0.95714286 0.97142857 0.98571429 1 1 1 1 1 1
  arc A34 (22.4846, -0.8319) -> (22.4846, 0.8319) centre (0, 0) ccw
  spline S17 degree 5 poles (22.4846, 0.8319) (22.4741, 0.8383) (22.453, 0.8511) (22.4214, 0.8701) (22.3791, 0.8953) (22.3263, 0.9265) (22.2733, 0.9573) (22.2203, 0.9878) (22.1672, 1.018) (22.114, 1.0479) (22.0608, 1.0775) (22.0075, 1.1067) (21.9541, 1.1356) (21.9007, 1.1642) (21.8471, 1.1925) (21.7936, 1.2204) (21.7399, 1.248) (21.6862, 1.2752) (21.6324, 1.3021) (21.5786, 1.3287) (21.5247, 1.3549) (21.4707, 1.3808) (21.4167, 1.4063) (21.3626, 1.4315) (21.3085, 1.4563) (21.2543, 1.4807) (21.2001, 1.5048) (21.1458, 1.5285) (21.0914, 1.5519) (21.037, 1.5749) (20.9826, 1.5975) (20.9281, 1.6198) (20.8736, 1.6416) (20.819, 1.6631) (20.7643, 1.6842) (20.7097, 1.7049) (20.655, 1.7252) (20.6002, 1.7451) (20.5454, 1.7646) (20.4906, 1.7837) (20.4357, 1.8024) (20.3808, 1.8206) (20.3259, 1.8384) (20.2709, 1.8558) (20.2159, 1.8728) (20.1609, 1.8893) (20.1059, 1.9054) (20.0508, 1.921) (19.9957, 1.9362) (19.9406, 1.9509) (19.8855, 1.9652) (19.8303, 1.9789) (19.7752, 1.9921) (19.72, 2.0048) (19.6648, 2.0169) (19.6096, 2.0285) (19.5544, 2.0396) (19.4992, 2.0503) (19.444, 2.0605) (19.3888, 2.0701) (19.3336, 2.079) (19.2784, 2.0871) (19.2232, 2.0944) (19.1681, 2.1008) (19.113, 2.1064) (19.0579, 2.1115) (19.0028, 2.1162) (18.9478, 2.1205) (18.8928, 2.1242) (18.8378, 2.1268) (18.783, 2.1276) (18.7393, 2.1263) (18.7065, 2.124) (18.6847, 2.1219) (18.6738, 2.1207) knots -1 -1 -1 -1 -1 -1 -0.98571429 -0.97142857 -0.95714286 -0.94285714 -0.92857143 -0.91428571 -0.9 -0.88571429 -0.87142857 -0.85714286 -0.84285714 -0.82857143 -0.81428571 -0.8 -0.78571429 -0.77142857 -0.75714286 -0.74285714 -0.72857143 -0.71428571 -0.7 -0.68571429 -0.67142857 -0.65714286 -0.64285714 -0.62857143 -0.61428571 -0.6 -0.58571429 -0.57142857 -0.55714286 -0.54285714 -0.52857143 -0.51428571 -0.5 -0.48571429 -0.47142857 -0.45714286 -0.44285714 -0.42857143 -0.41428571 -0.4 -0.38571429 -0.37142857 -0.35714286 -0.34285714 -0.32857143 -0.31428571 -0.3 -0.28571429 -0.27142857 -0.25714286 -0.24285714 -0.22857143 -0.21428571 -0.2 -0.18571429 -0.17142857 -0.15714286 -0.14285714 -0.12857143 -0.11428571 -0.1 -0.08571429 -0.07142857 -0.05714286 -0.04285714 -0.02857143 -0.01428571 0 0 0 0 0 0
  line L17 (18.6738, 2.1207) -> (17.8062, 2.0227)
  arc A35 (16.7082, 2.8483) -> (17.8062, 2.0227) centre (17.6939, 3.0163) ccw
  arc A36 (16.7082, 2.8483) -> (16.5263, 3.7625) centre (0, 0) ccw
  arc A37 (17.2248, 4.9454) -> (16.5263, 3.7625) centre (17.5014, 3.9844) ccw
  line L18 (17.2248, 4.9454) -> (18.0639, 5.1869)
  spline S18 degree 5 poles (18.0639, 5.1869) (18.0744, 5.19) (18.0954, 5.1963) (18.1265, 5.2067) (18.1674, 5.2223) (18.2178, 5.2441) (18.2675, 5.2675) (18.3169, 5.2919) (18.3661, 5.3169) (18.4152, 5.3423) (18.4642, 5.3681) (18.5129, 5.3944) (18.5614, 5.4215) (18.6096, 5.4493) (18.6575, 5.4779) (18.7051, 5.5073) (18.7524, 5.5373) (18.7995, 5.5678) (18.8464, 5.5988) (18.8932, 5.6302) (18.9397, 5.662) (18.9861, 5.6944) (19.0322, 5.7272) (19.0781, 5.7605) (19.1238, 5.7942) (19.1693, 5.8285) (19.2146, 5.8632) (19.2597, 5.8983) (19.3046, 5.9338) (19.3493, 5.9698) (19.3938, 6.0061) (19.4381, 6.0428) (19.4822, 6.0799) (19.5261, 6.1174) (19.5699, 6.1552) (19.6134, 6.1935) (19.6568, 6.2321) (19.6999, 6.2711) (19.7429, 6.3105) (19.7857, 6.3502) (19.8283, 6.3902) (19.8707, 6.4306) (19.9129, 6.4713) (19.9549, 6.5124) (19.9967, 6.5538) (20.0384, 6.5955) (20.0798, 6.6376) (20.1211, 6.68) (20.1622, 6.7227) (20.2031, 6.7657) (20.2438, 6.809) (20.2843, 6.8526) (20.3246, 6.8966) (20.3648, 6.9408) (20.4047, 6.9854) (20.4445, 7.0302) (20.484, 7.0754) (20.5234, 7.1208) (20.5626, 7.1665) (20.6016, 7.2125) (20.6405, 7.2588) (20.6791, 7.3054) (20.7175, 7.3523) (20.7558, 7.3994) (20.7939, 7.4468) (20.8317, 7.4945) (20.8694, 7.5425) (20.9069, 7.5907) (20.9442, 7.6392) (20.9813, 7.688) (21.0182, 7.737) (21.0476, 7.7764) (21.0696, 7.8061) (21.0842, 7.8259) (21.0914, 7.8359) knots 0 0 0 0 0 0 0.01428571 0.02857143 0.04285714 0.05714286 0.07142857 0.08571429 0.1 0.11428571 0.12857143 0.14285714 0.15714286 0.17142857 0.18571429 0.2 0.21428571 0.22857143 0.24285714 0.25714286 0.27142857 0.28571429 0.3 0.31428571 0.32857143 0.34285714 0.35714286 0.37142857 0.38571429 0.4 0.41428571 0.42857143 0.44285714 0.45714286 0.47142857 0.48571429 0.5 0.51428571 0.52857143 0.54285714 0.55714286 0.57142857 0.58571429 0.6 0.61428571 0.62857143 0.64285714 0.65714286 0.67142857 0.68571429 0.7 0.71428571 0.72857143 0.74285714 0.75714286 0.77142857 0.78571429 0.8 0.81428571 0.82857143 0.84285714 0.85714286 0.87142857 0.88571429 0.9 0.91428571 0.92857143 0.94285714 0.95714286 0.97142857 0.98571429 1 1 1 1 1 1
  arc A38 (21.0914, 7.8359) -> (20.4547, 9.3731) centre (0, 0) ccw
  spline S19 degree 5 poles (20.4547, 9.3731) (20.4425, 9.375) (20.4182, 9.3787) (20.3817, 9.3842) (20.333, 9.3913) (20.2722, 9.3998) (20.2115, 9.4081) (20.1508, 9.416) (20.0902, 9.4236) (20.0297, 9.4308) (19.9692, 9.4378) (19.9087, 9.4444) (19.8484, 9.4507) (19.788, 9.4566) (19.7278, 9.4622) (19.6676, 9.4675) (19.6075, 9.4725) (19.5474, 9.4771) (19.4874, 9.4814) (19.4275, 9.4853) (19.3677, 9.4889) (19.308, 9.4922) (19.2483, 9.4951) (19.1887, 9.4976) (19.1292, 9.4998) (19.0698, 9.5017) (19.0104, 9.5032) (18.9512, 9.5043) (18.8921, 9.5051) (18.833, 9.5055) (18.774, 9.5056) (18.7152, 9.5053) (18.6564, 9.5046) (18.5978, 9.5036) (18.5392, 9.5021) (18.4808, 9.5003) (18.4225, 9.4982) (18.3643, 9.4956) (18.3062, 9.4926) (18.2482, 9.4893) (18.1904, 9.4856) (18.1327, 9.4814) (18.0751, 9.4769) (18.0177, 9.4719) (17.9604, 9.4665) (17.9033, 9.4607) (17.8462, 9.4545) (17.7894, 9.4479) (17.7327, 9.4409) (17.6761, 9.4334) (17.6197, 9.4254) (17.5635, 9.417) (17.5075, 9.4081) (17.4517, 9.3987) (17.3961, 9.3887) (17.3406, 9.3784) (17.2854, 9.3675) (17.2303, 9.3563) (17.1754, 9.3445) (17.1207, 9.3323) (17.0663, 9.3194) (17.0122, 9.3058) (16.9585, 9.2914) (16.9051, 9.2762) (16.852, 9.2603) (16.7991, 9.2439) (16.7465, 9.2272) (16.694, 9.2101) (16.6417, 9.1924) (16.59, 9.1738) (16.539, 9.1536) (16.4991, 9.1357) (16.4697, 9.121) (16.4504, 9.1107) (16.4408, 9.1054) knots -1 -1 -1 -1 -1 -1 -0.98571429 -0.97142857 -0.95714286 -0.94285714 -0.92857143 -0.91428571 -0.9 -0.88571429 -0.87142857 -0.85714286 -0.84285714 -0.82857143 -0.81428571 -0.8 -0.78571429 -0.77142857 -0.75714286 -0.74285714 -0.72857143 -0.71428571 -0.7 -0.68571429 -0.67142857 -0.65714286 -0.64285714 -0.62857143 -0.61428571 -0.6 -0.58571429 -0.57142857 -0.55714286 -0.54285714 -0.52857143 -0.51428571 -0.5 -0.48571429 -0.47142857 -0.45714286 -0.44285714 -0.42857143 -0.41428571 -0.4 -0.38571429 -0.37142857 -0.35714286 -0.34285714 -0.32857143 -0.31428571 -0.3 -0.28571429 -0.27142857 -0.25714286 -0.24285714 -0.22857143 -0.21428571 -0.2 -0.18571429 -0.17142857 -0.15714286 -0.14285714 -0.12857143 -0.11428571 -0.1 -0.08571429 -0.07142857 -0.05714286 -0.04285714 -0.02857143 -0.01428571 0 0 0 0 0 0
  line L19 (16.4408, 9.1054) -> (15.6767, 8.6828)
  arc A39 (14.3463, 9.0254) -> (15.6767, 8.6828) centre (15.1928, 9.5579) ccw
  arc A40 (14.3463, 9.0254) -> (13.8285, 9.8004) centre (0, 0) ccw
  arc A41 (14.0211, 11.1606) -> (13.8285, 9.8004) centre (14.6444, 10.3786) ccw
  line L20 (14.0211, 11.1606) -> (14.7039, 11.7048)